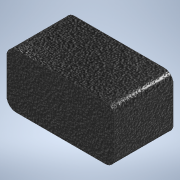
# Autodesk Inventor part: BatteryV1
Saved by Autodesk Inventor 2020 (Build 240168000, 168)
## iProperties
Created: 2023-11-25
Part Number: BatteryV1
Material: Generic
Document SubType Name: Modeling
Designer: smz3rm
Density: 1.60879 g/cm^3
Appearance: Default
Mass: 42 g
Surface Area: 53.6685 cm^2
Volume: 26.1066 cm^3
Author: smz3rm
Autodesk Inventor part; units mm, degrees
ref_plane "YZ Plane" through (0, 0, 0) normal (1, 0, 0) x (0, 1, 0)
ref_plane "XZ Plane" through (0, 0, 0) normal (0, 1, 0) x (-1, 0, 0)
ref_plane "XY Plane" through (0, 0, 0) normal (0, 0, 1) x (1, 0, 0)
sketch "Sketch1" plane through (0, 0, 0) normal (0, 1, 0) x (-1, 0, 0)
  line L0 (23, 12.5) -> (-23, 12.5)
  line L1 (-23, 12.5) -> (-23, -12.5)
  line L2 (-23, -12.5) -> (23, -12.5)
  line L3 (23, -12.5) -> (23, 12.5)
  line L4 (23, 12.5) -> (-23, -12.5) construction
  line L5 (-23, 12.5) -> (23, -12.5) construction
  point P0 (0, 0)
  dimension "d0" = 46
  dimension "d1" = 25
  constraints: 12 end point, 2 midpoint, 2 parallel, 1 horizontal, 1 perpendicular
  measures "d0" distance of L2.end L1.end
  measures "d1" distance of L0.end L1.end
extrude "Extrusion1" add sketch "Sketch1" along normal blind 23
fillet "Fillet1" radius 4 4 edges at (23, 23, 0) (23, 0, 0) (-23, 23, 0) (-23, 0, 0)
body "Solid1"
